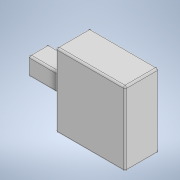
# Autodesk Inventor part: dual_slider_paddlew
Saved by Autodesk Inventor 2022 (Build 260153000, 153)
## iProperties
Created: 2022-03-29
Part Number: dual_slider_paddlew
Material: Generic
Document SubType Name: Modeling
Designer: thoms
Density: 1 g/cm^3
Appearance: Default
Author: thoms
Autodesk Inventor part; units mm, degrees
ref_plane "YZ Plane" through (0, 0, 0) normal (1, 0, 0) x (0, 1, 0)
ref_plane "XZ Plane" through (0, 0, 0) normal (0, 1, 0) x (-1, 0, 0)
ref_plane "XY Plane" through (0, 0, 0) normal (0, 0, 1) x (1, 0, 0)
sketch "Sketch1" plane through (0, 0, 0) normal (1, 0, 0) x (0, 1, 0)
  line L0 (1.325, 1.45) -> (-1.325, 1.45)
  line L1 (-1.325, 1.45) -> (-1.325, -1.45)
  line L2 (-1.325, -1.45) -> (1.325, -1.45)
  line L3 (1.325, -1.45) -> (1.325, 1.45)
  point P0 (0, 0)
  dimension "d0" = 2.9
  dimension "d1" = 2.65
  dimension "d2" = 1.45
  dimension "d3" = 1.325
  constraints: 8 end point, 2 parallel, 1 horizontal, 1 perpendicular
  measures "d0" distance of L2.end L0.start
  measures "d1" distance of L1.end L2.end
  measures "d2" distance from line of point (0, 0) L0
  measures "d3" distance from line of point (0, 0) L1
extrude "Extrusion1" add sketch "Sketch1" against normal blind 5
sketch "Sketch2" plane through (0, 0, 0) normal (1, 0, 0) x (0, 0, -1)
  line L0 (-2.45, 5.325) -> (2.45, 5.325)
  line L1 (2.45, 5.325) -> (2.45, -5.325)
  line L2 (2.45, -5.325) -> (-2.45, -5.325)
  line L3 (-2.45, -5.325) -> (-2.45, 5.325)
  line L4 (-1.45, 1.325) -> (-1.45, -1.325) projected
  line L5 (1.45, -1.325) -> (1.45, 1.325) projected
  line L6 (1.45, 1.325) -> (-1.45, 1.325) projected
  line L7 (-1.45, -1.325) -> (1.45, -1.325) projected
  point P0 (0, 0)
  dimension "d6" = 1
  dimension "d7" = 1
  dimension "d8" = 4
  dimension "d9" = 4
  constraints: 8 end point, 2 parallel, 1 horizontal, 1 perpendicular
  measures "d6" distance between parallel lines of L4 L3
  measures "d7" distance between parallel lines of L1 L5
  measures "d8" distance between parallel lines of L0 L6
  measures "d9" distance between parallel lines of L7 L2
extrude "Extrusion2" add sketch "Sketch2" along normal blind 10 contours L0 L1 L2 L3 | L6 L5 L7 L4
fillet "Fillet1" radius 0.25 24 edges at (5, 5.325, 2.45) (5, 5.325, -2.45) (5, -5.325, -2.45) (5, -5.325, 2.45) (10, -5.325, 0) (10, 0, 2.45) (10, 0, -2.45) (10, 5.325, 0) (0, 5.325, 0) (0, -5.325, 0) (0, 0, 2.45) (0, 0, -2.45) (-2.5, 1.325, -1.45) (-2.5, 1.325, 1.45) (-2.5, -1.325, -1.45) (-2.5, -1.325, 1.45) (0, 1.325, 0) (0, 0, 1.45) (0, 0, -1.45) (0, -1.325, 0) (-5, 0, 1.45) (-5, 1.325, 0) (-5, 0, -1.45) (-5, -1.325, 0)
body "Solid1"
